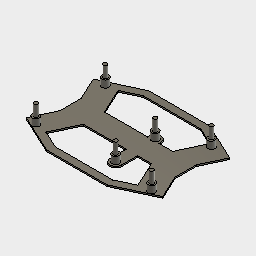
Arduino Mount V1.0 v7 (Autodesk Fusion 360 design; units mm, degrees)
Autodesk Fusion 360 part; units mm, degrees
sketch "Sketch1" plane through (0, 0, 0) normal (0, 1, 0) x (1, 0, 0)
  line L0 (13.8907, 50.6995) -> (18.8907, 50.6995) construction
  line L1 (13.8907, 50.6995) -> (21.3907, 50.6995) construction
  line L2 (21.5332, 52.0565) -> (29.9066, 34.0997)
  line L3 (13.8907, 50.6995) -> (21.3907, 50.6995) construction
  line L4 (7.0934, 47.5298) -> (13.3559, 34.0997)
  line L5 (7.0934, 5.6696) -> (13.3559, 19.0997)
  line L6 (21.5332, 1.143) -> (29.9066, 19.0997)
  line L7 (7.0934, 47.5298) -> (5.8255, 50.2488)
  line L8 (7.0934, 47.5298) -> (12.0934, 47.5298) construction
  line L9 (7.0934, 5.6696) -> (5.8255, 2.9507)
  line L10 (7.0934, 5.6696) -> (12.0934, 5.6696) construction
  line L11 (4.9803, 1.1381) -> (19.9803, 1.1381) construction
  line L12 (13.3559, 34.0997) -> (13.3559, 19.0997)
  line L13 (96.6149, 2.5) -> (104.1149, 2.5) construction
  line L14 (85.1097, 49.1342) -> (78.099, 34.0997)
  line L15 (86.4724, 1.143) -> (78.099, 19.0997)
  line L16 (94.6496, 34.0997) -> (94.6496, 19.0997)
  line L17 (100.9122, 5.6696) -> (94.6496, 19.0997)
  line L18 (100.9122, 47.5298) -> (94.6496, 34.0997)
  line L19 (100.9122, 47.5298) -> (102.1801, 50.2488)
  line L20 (100.9122, 5.6696) -> (102.3902, 2.5)
  line L21 (29.9066, 34.0997) -> (60.3566, 34.0997)
  line L22 (68.3041, 34.0997) -> (78.099, 34.0997)
  arc A0 (68.3041, 35.3466) -> (60.3097, 35.3466) centre (64.3069, 35.4968) ccw
  line L23 (60.3097, 7.4466) -> (60.3097, 19.0997)
  line L24 (68.3069, 7.5968) -> (68.3069, 19.0997)
  arc A1 (60.3097, 7.747) -> (68.3069, 7.5968) centre (64.3069, 7.5968) ccw
  line L25 (29.9066, 19.0997) -> (60.3097, 19.0997)
  line L26 (68.3069, 19.0997) -> (78.099, 19.0997)
  line L27 (60.3097, 35.3466) -> (60.3566, 34.0997)
  line L28 (68.3041, 35.3466) -> (68.3041, 34.0989)
  line L29 (85.1097, 49.1342) -> (86.4724, 52.0565)
  line L30 (89.4307, -5.2012) -> (104.4307, -5.2012) construction
  line L31 (89.4307, -5.2012) -> (96.4307, -5.2012) construction
  line L32 (18.5749, -5.2012) -> (25.5749, -5.2012) construction
  line L33 (54.0028, -4.5404) -> (33.7214, -4.5404)
  line L34 (33.7214, -4.5404) -> (54.0028, -4.5404)
  line L35 (54.0028, -4.5404) -> (74.2842, -4.5404)
  line L36 (21.5332, 1.143) -> (33.7214, -4.5404)
  line L37 (21.5332, 1.143) -> (36.7862, 1.143) construction
  line L38 (86.4724, 1.143) -> (74.2842, -4.5404)
  line L39 (86.4724, 1.143) -> (101.7194, 1.143) construction
  line L40 (21.5332, 52.0565) -> (33.7214, 57.7399)
  line L41 (54.0028, 57.7399) -> (33.7214, 57.7399)
  line L42 (54.0028, 57.7399) -> (74.2842, 57.7399)
  line L43 (86.4724, 52.0565) -> (74.2842, 57.7399)
  line L44 (4.9803, 1.1381) -> (6.9803, 1.1381) construction
  line L45 (102.3902, 2.5) -> (102.1801, 2.9507)
  line L46 (102.1801, 2.9507) -> (75.3927, -9.5404)
  line L47 (5.8255, 2.9507) -> (32.6129, -9.5404)
  line L48 (54.0028, -9.5404) -> (75.3927, -9.5404)
  line L49 (54.0028, -9.5404) -> (32.6129, -9.5404)
  line L50 (13.3559, 26.5997) -> (94.6496, 26.5997)
  line L51 (5.8255, 50.2488) -> (32.6129, 62.7399)
  line L52 (54.0028, 62.7399) -> (32.6129, 62.7399)
  line L53 (102.1801, 50.2488) -> (75.3927, 62.7399)
  line L54 (54.0028, 62.7399) -> (75.3927, 62.7399)
  dimension "d15" = 27.9
  dimension "d91" = 7.5
  dimension "d95" = 115
  dimension "d97" = 115
  dimension "d98" = 5
  dimension "d100" = 15
  dimension "d107" = 8
  dimension "d109" = 8
  dimension "d110" = 1.2478
  dimension "d224" = 7
  dimension "d227" = 7
  dimension "d228" = 25
  dimension "d230" = 155
  dimension "d249" = 2
  constraint horizontal L0
  constraint horizontal L1
  constraint horizontal L3
  constraint horizontal L8
  constraint horizontal L10
  constraint horizontal L11
  constraint horizontal L21
  constraint horizontal L13
  constraint collinear L21 L22
  constraint coincident A1
  constraint perpendicular L23 L25
  constraint coincident origin L25
  constraint tangent L24 A1
  constraint perpendicular L24 L25
  constraint coincident L23
  constraint collinear L25 L26
  constraint tangent A0 L27
  constraint vertical L28
  constraint coincident L28
  constraint parallel L14 L29
  constraint horizontal L30
  constraint horizontal L31
  constraint horizontal L32
  constraint horizontal L37
  constraint horizontal L39
  constraint horizontal L44
  constraint coincident L20 origin
  constraint parallel L20 L45
  constraint perpendicular L45 L46
  constraint midpoint L12
  constraint midpoint L16
  constraint perpendicular L16 L50
  constraint coincident L13 origin
  measures "d91" distance of origin
  measures "d95" angle of L7 L8
  measures "d97" angle of L9 L10
  measures "d98" distance of origin
  measures "d107" diameter of A0
  measures "d109" diameter of A1
  measures "d110" distance of origin
  measures "d228" angle of L36 L37
  measures "d230" angle of L38 L39
  measures "d249" distance of origin
extrude "Extrude1" add sketch "Sketch1" along normal blind 1
sketch "Sketch27" plane through (0, 1, 0) normal (0, 1, 0) x (-1, 0, 0)
  line L0 (-60.3097, -19.0997) -> (-60.3097, -7.4466)
  arc A0 (-60.3097, -7.4466) -> (-68.3069, -7.5968) centre (-64.3069, -7.5968) ccw
  line L1 (-68.3069, -7.5968) -> (-68.3069, -19.0997)
  line L2 (-68.3069, -19.0997) -> (-78.099, -19.0997)
  line L3 (-78.099, -19.0997) -> (-86.4724, -1.143)
  line L4 (-86.4724, -1.143) -> (-74.2842, 4.5404)
  line L5 (-74.2842, 4.5404) -> (-33.7214, 4.5404)
  line L6 (-33.7214, 4.5404) -> (-21.5332, -1.143)
  line L7 (-21.5332, -1.143) -> (-29.9066, -19.0997)
  line L8 (-29.9066, -19.0997) -> (-60.3097, -19.0997)
  line L9 (-86.4724, -52.0565) -> (-78.099, -34.0997)
  line L10 (-78.099, -34.0997) -> (-68.3041, -34.0997)
  line L11 (-68.3041, -34.0997) -> (-68.3041, -35.3466)
  arc A1 (-68.3041, -35.3466) -> (-60.3097, -35.3466) centre (-64.3069, -35.4968) ccw
  line L12 (-60.3097, -35.3466) -> (-60.3566, -34.0997)
  line L13 (-60.3566, -34.0997) -> (-29.9066, -34.0997)
  line L14 (-29.9066, -34.0997) -> (-21.5332, -52.0565)
  line L15 (-21.5332, -52.0565) -> (-33.7214, -57.7399)
  line L16 (-33.7214, -57.7399) -> (-74.2842, -57.7399)
  line L17 (-74.2842, -57.7399) -> (-86.4724, -52.0565)
  line L18 (-94.6496, -34.0997) -> (-102.1801, -50.2488)
  line L19 (-5.8255, -50.2488) -> (-13.3559, -34.0997)
  line L20 (-13.3559, -34.0997) -> (-13.3559, -19.0997)
  line L21 (-13.3559, -19.0997) -> (-5.8255, -2.9507)
  line L22 (-102.1801, -2.9507) -> (-94.6496, -19.0997)
  line L23 (-94.6496, -19.0997) -> (-94.6496, -34.0997)
  circle A2 centre (-13.1007, -2.4428) radius 2.5
  circle A3 centre (-13.8907, -50.6995) radius 2.5
  circle A4 centre (-64.3069, -35.4968) radius 2.5
  circle A5 centre (-64.3069, -7.5968) radius 2.5
  circle A6 centre (-94.9048, -2.4428) radius 2.5
  circle A7 centre (-88.7907, -50.6995) radius 2.5
  line L24 (-5.8255, -2.9507) -> (-32.6129, 9.5404)
  line L25 (-32.6129, 9.5404) -> (-75.3927, 9.5404)
  line L26 (-75.3927, 9.5404) -> (-102.1801, -2.9507)
  line L27 (-102.1801, -50.2488) -> (-75.3927, -62.7399)
  line L28 (-75.3927, -62.7399) -> (-32.6129, -62.7399)
  line L29 (-32.6129, -62.7399) -> (-5.8255, -50.2488)
  dimension "d232" = 5
  dimension "d233" = 5
  dimension "d234" = 5
  dimension "d235" = 5
  dimension "d236" = 5
  dimension "d237" = 5
  measures "d232" diameter of A2
  measures "d233" diameter of A3
  measures "d234" diameter of A4
  measures "d235" diameter of A5
  measures "d236" diameter of A6
  measures "d237" diameter of A7
extrude "Extrude17" add sketch "Sketch27" along normal blind 5 and the other way blind 1 contours A2 | A3 | A4 | A5 | A6 | A7
ref_plane "WorkPlane2" through (54.0028, 6, -26.5997) normal (0, 1, 0) x (1, 0, 0)
sketch "Sketch29" plane through (54.0028, 6, -26.5997) normal (0, 1, 0) x (1, 0, 0)
  circle A0 centre (-40.1121, 24.0997) radius 2.5
  circle A1 centre (10.3041, 8.8971) radius 2.5
  circle A2 centre (34.7879, 24.0997) radius 2.5
  circle A3 centre (40.9021, -24.1569) radius 2.5
  circle A4 centre (10.3041, -19.0029) radius 2.5
  circle A5 centre (-40.9021, -24.1569) radius 2.5
  circle A6 centre (-40.1121, 24.0997) radius 1.4
  circle A7 centre (-40.9021, -24.1569) radius 1.4
  circle A8 centre (10.3041, -19.0029) radius 1.4
  circle A9 centre (40.9021, -24.1569) radius 1.4
  circle A10 centre (10.3041, 8.8971) radius 1.4
  circle A11 centre (34.7879, 24.0997) radius 1.4
  dimension "d254" = 2.8
  dimension "d255" = 2.8
  dimension "d256" = 2.8
  dimension "d257" = 2.8
  dimension "d258" = 2.8
  dimension "d259" = 2.8
  constraint concentric A0 A6
  constraint concentric A5 A7
  constraint concentric A4 A8
  constraint concentric A3 A9
  constraint concentric A1 A10
  constraint concentric A2 A11
  measures "d254" diameter of A6
  measures "d255" diameter of A7
  measures "d256" diameter of A8
  measures "d257" diameter of A9
  measures "d258" diameter of A10
  measures "d259" diameter of A11
extrude "Extrude19" add sketch "Sketch29" along normal blind 8 contours A6 | A7 | A8 | A9 | A10 | A11
